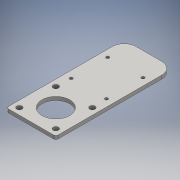
# Autodesk Inventor part: body1
Saved by Autodesk Inventor 2016 SP1 (Build 200210100, 210)
## iProperties
Created: 2018-04-30
Part Number: body1
Material: 一般
Document SubType Name: Modeling
Designer: kobay
Density: 1 g/cm^3
Appearance: 既定
Author: kobay
Autodesk Inventor part; units mm, degrees
ref_plane "YZ Plane" through (0, 0, 0) normal (1, 0, 0) x (0, 1, 0)
ref_plane "XZ Plane" through (0, 0, 0) normal (0, 1, 0) x (-1, 0, 0)
ref_plane "XY Plane" through (0, 0, 0) normal (0, 0, 1) x (1, 0, 0)
sketch "スケッチ1" plane through (0, 0, 0) normal (0, 0, 1) x (1, 0, 0)
  line L0 (0, 0) -> (42, 0)
  line L1 (42, 0) -> (42, 100)
  line L2 (42, 100) -> (0, 100)
  line L3 (0, 100) -> (0, 0)
  line L4 (0, 42) -> (42, 42)
  circle A0 centre (5.5, 36.5) radius 2.25
  circle A1 centre (36.5, 36.5) radius 2.25
  circle A2 centre (5.5, 5.5) radius 2.25
  circle A3 centre (36.5, 5.5) radius 2.25
  circle A4 centre (21, 21) radius 11.75
  dimension "d0" = 42
  dimension "d1" = 100
  dimension "d2" = 42
  dimension "d3" = 5.5
  dimension "d4" = 5.5
  dimension "d5" = 5.5
  dimension "d6" = 5.5
  dimension "d7" = 4.5
  dimension "d8" = 4.5
  dimension "d9" = 4.5
  dimension "d10" = 4.5
  dimension "d11" = 23.5
  constraints: 10 end point, 5 centre point, 4 coincident, 2 parallel, 2 perpendicular, 2 point on line, 1 horizontal
  measures "d0" distance of L2.end L1.end
  measures "d1" distance of L1.end L0.end
  measures "d2" distance between parallel lines of L0 L4
  measures "d3" distance from line of L0 point (36.5, 5.5)
  measures "d4" distance from line of L1 point (36.5, 5.5)
  measures "d5" distance from line of point (36.5, 36.5) L4
  measures "d6" distance from line of point (5.5, 36.5) L3
  measures "d7" diameter of A0
  measures "d8" diameter of A1
  measures "d9" diameter of A2
  measures "d10" diameter of A3
  measures "d11" diameter of A4
extrude "押し出し1" add sketch "スケッチ1" along normal blind 3
fillet "フィレット1" radius 2 2 edges at (42, 0, 1.5) (0, 0, 1.5)
fillet "フィレット2" radius 10 2 edges at (0, 100, 1.5) (42, 100, 1.5)
sketch "スケッチ2" plane through (0, 0, 3) normal (0, 0, 1) x (1, 0, 0)
  line L0 (0, 90) -> (0, 2) projected
  line L1 (0, 46) -> (42, 46)
  line L2 (42, 2) -> (42, 90) projected
  line L3 (0, 52) -> (42, 52)
  line L4 (6, 52) -> (6, 46)
  line L5 (36, 52) -> (36, 46)
  circle A0 centre (6, 49) radius 1.3
  circle A1 centre (36, 49) radius 1.3
  point P0 (0, 0)
  dimension "d16" = 6
  dimension "d17" = 6
  dimension "d18" = 6
  dimension "d19" = 2.6
  dimension "d20" = 2.6
  constraints: 8 end point, 6 point on line, 4 midpoint, 2 centre point, 2 perpendicular, 1 parallel
  measures "d16" distance between parallel lines of L3 L1
  measures "d17" distance between parallel lines of L4 L0
  measures "d18" distance between parallel lines of L2 L5
  measures "d19" diameter of A0
  measures "d20" diameter of A1
extrude "押し出し2" cut sketch "スケッチ2" against normal blind 3 contours A0 L4 | L4 A0 | A1 L5 | L5 A1
sketch "スケッチ3" plane through (0, 0, 3) normal (0, 0, 1) x (1, 0, 0)
  line L0 (0, 90) -> (0, 2)
  line L1 (0, 46) -> (42, 46)
  line L2 (42, 2) -> (42, 90)
  line L3 (0, 52) -> (42, 52)
  line L4 (6, 52) -> (6, 46)
  line L5 (36, 52) -> (36, 46)
  circle A0 centre (6, 49) radius 1.3
  circle A1 centre (36, 49) radius 1.3
  line L6 (0, 90) -> (0, 2) projected
  line L7 (0, 77) -> (42, 77)
  line L8 (42, 2) -> (42, 90) projected
  line L9 (0, 83) -> (42, 83)
  circle A2 centre (6, 80) radius 1.3
  circle A3 centre (36, 80) radius 1.3
  point P0 (0, 0)
  point P1 (0, 0)
  dimension "d23" = 6
  dimension "d24" = 6
  dimension "d25" = 6
  dimension "d26" = 2.6
  dimension "d27" = 2.6
  dimension "d28" = 25
  dimension "d29" = 6
  dimension "d30" = 2.6
  dimension "d31" = 3
  dimension "d32" = 2.6
  constraints: 16 end point, 10 point on line, 4 centre point, 4 midpoint, 3 perpendicular, 1 horizontal, 1 parallel
  measures "d23" distance between parallel lines of L3 L1
  measures "d24" distance between parallel lines of L4 L0
  measures "d25" distance between parallel lines of L2 L5
  measures "d26" diameter of A0
  measures "d27" diameter of A1
  measures "d28" distance between parallel lines of L3 L7
  measures "d29" distance between parallel lines of L7 L9
  measures "d30" diameter of A2
  measures "d31" distance from line of A2.centre L9
  measures "d32" diameter of A3
extrude "押し出し3" cut sketch "スケッチ3" against normal blind 10 contours A2 | A3
